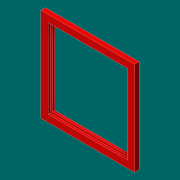
# Autodesk Inventor part: aerogelHolder
Saved by Autodesk Inventor 2016 (Build 200138000, 138)
## iProperties
Created: 2015-10-27
Part Number: aerogelHolder
Material: ABS Plastic
Document SubType Name: Modeling
Designer: Sawaiz
Density: 1.06 g/cm^3
Appearance: Smooth - Red
Author: Sawaiz
Autodesk Inventor part; units mm, degrees
ref_plane "YZ Plane" through (0, 0, 0) normal (1, 0, 0) x (0, 1, 0)
ref_plane "XZ Plane" through (0, 0, 0) normal (0, 1, 0) x (-1, 0, 0)
ref_plane "XY Plane" through (0, 0, 0) normal (0, 0, 1) x (1, 0, 0)
sketch "Sketch1" plane through (0, 0, 0) normal (1, 0, 0) x (0, 1, 0)
  line L0 (-66.675, -66.675) -> (66.675, -66.675)
  line L1 (66.675, -66.675) -> (66.675, 66.675)
  line L2 (66.675, 66.675) -> (-66.675, 66.675)
  line L3 (-66.675, 66.675) -> (-66.675, -66.675)
  line L4 (-66.675, -66.675) -> (66.675, 66.675) construction
  line L5 (66.675, -66.675) -> (-66.675, 66.675) construction
  point P0 (0, 0)
  dimension "d0" = 133.35
  dimension "d1" = 133.35
  constraints: 12 end point, 2 midpoint, 2 parallel, 1 horizontal, 1 perpendicular
  measures "d0" distance of L2.end L1.end
  measures "d1" distance of L1.end L0.end
extrude "Extrusion1" add sketch "Sketch1" along normal blind 6.35
sketch "Sketch2" plane through (6.35, 0, 0) normal (1, 0, 0) x (0, 0, -1)
  line L0 (56.5875, -56.5875) -> (-56.5875, -56.5875)
  line L1 (-56.5875, -56.5875) -> (-56.5875, 56.5875)
  line L2 (-56.5875, 56.5875) -> (56.5875, 56.5875)
  line L3 (56.5875, 56.5875) -> (56.5875, -56.5875)
  line L4 (56.5875, -56.5875) -> (-56.5875, 56.5875) construction
  line L5 (-56.5875, -56.5875) -> (56.5875, 56.5875) construction
  point P0 (0, 0)
  dimension "d4" = 113.175
  dimension "d5" = 113.175
  constraints: 12 end point, 2 midpoint, 2 parallel, 1 horizontal, 1 perpendicular
  measures "d4" distance of L1.end L2.end
  measures "d5" distance of L0.end L1.end
extrude "Extrusion2" cut sketch "Sketch2" against normal blind 3.175
sketch "Sketch3" plane through (3.175, 0, 0) normal (1, 0, 0) x (0, 0, -1)
  line L0 (56.5875, -56.5875) -> (-56.5875, -56.5875) projected
  line L1 (56.5875, 56.5875) -> (56.5875, -56.5875) projected
  line L2 (-56.5875, 56.5875) -> (56.5875, 56.5875) projected
  line L3 (-56.5875, -56.5875) -> (-56.5875, 56.5875) projected
  line L4 (-53.4125, 53.4125) -> (53.4125, 53.4125)
  line L5 (53.4125, 53.4125) -> (53.4125, -53.4125)
  line L6 (53.4125, -53.4125) -> (-53.4125, -53.4125)
  line L7 (-53.4125, -53.4125) -> (-53.4125, 53.4125)
  point P0 (0, 0)
  dimension "d8" = 3.175
  constraints: 8 end point, 3 other
  measures "d8" distance between parallel lines of L3 L7
extrude "Extrusion3" cut sketch "Sketch3" against normal through all contours L4 L5 L6 L7
equation "\"d0\" = width + internalAcrylicThickness"
equation "\"d1\" = height + internalAcrylicThickness"
equation "\"d2\" = internalAcrylicThickness"
equation "\"d4\" = aerogelHeight + aerogelClearence"
equation "\"d5\" = aerogelWidth + aerogelClearence"
equation "\"d6\" = 0.5 * internalAcrylicThickness"
equation "\"d8\" = aerogelClearence"
equation "\"d9\" = 0.5 * internalAcrylicThickness"
equation "\"frameAcrylicThickness\" = 9.525"
equation "\"internalAcrylicThickness\" = 6.35"
equation "\"aerogelWidth\" = 110"
equation "\"aerogelHeight\" = 110"
equation "\"height\" = 127"
equation "\"width\" = 127"
equation "\"depth\" = 273.05"
equation "\"mirrorAngle\" = 5deg"
equation "\"detectorWidth\" = 52"
equation "\"detectorHeight\" = 52"
equation "\"mirrorThickness\" = 3.175"
equation "\"fresnelThickness\" = 0.1"
equation "\"focalLength\" = 76.2"
equation "\"ior\" = 1.49"
equation "\"centerThickness\" = 1.524"
equation "\"fresnelAngle\" = 90deg"
equation "\"fresnelEffectiveDiameter\" = 152.4"
equation "\"oRingWidth\" = 1.5875"
equation "\"sensorHolderDepth\" = 19.05"
equation "\"aerogelClearence\" = 3.175"
equation "\"backplanePostionOffsett\" = 12.7"
equation "\"backplaneHoleOffsett\" = 6.35"
equation "\"backplanePCBHeight\" = 76.2"
equation "\"backplanePCBWidth\" = 76.2"
equation "\"moduleSlotClearence\" = 0.79375"
body "Solid1"
